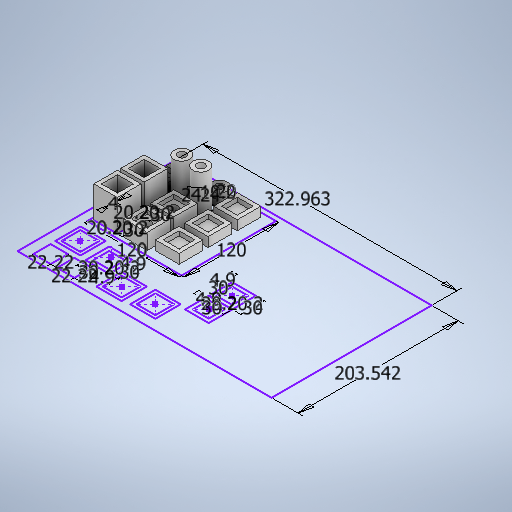
# Autodesk Inventor part: zxie2
Saved by Autodesk Inventor 2025.1 (Build 291241000, 241)
## iProperties
Created: 2024-10-25
Part Number: zxie2
Material: 一般
Document SubType Name: Modeling
Designer: youtian
Density: 1 g/cm^3
Appearance: 預設
Author: youtian
Autodesk Inventor part; units mm, degrees
ref_plane "YZ Plane" through (0, 0, 0) normal (1, 0, 0) x (0, 1, 0)
ref_plane "XZ Plane" through (0, 0, 0) normal (0, 1, 0) x (-1, 0, 0)
ref_plane "XY Plane" through (0, 0, 0) normal (0, 0, 1) x (1, 0, 0)
sketch "草圖1" plane through (0, 0, 0) normal (0, 1, 0) x (-1, 0, 0)
  circle A0 centre (0, 0) radius 5.1
  circle A1 centre (0, 0) radius 10
  line L0 (0, 0) -> (-26.517, 0)
  line L1 (0, 0) -> (0, 28.4195)
  circle A2 centre (-24, 0) radius 5.1
  circle A3 centre (-24, 0) radius 10
  circle A4 centre (0, 24) radius 5.1
  circle A5 centre (0, 24) radius 10
  circle A6 centre (-24, 24) radius 5.1
  circle A7 centre (-24, 24) radius 10
  dimension "d6" = 24
  dimension "d9" = 24
  dimension "d137" = 10.2
  dimension "d138" = 20
  constraints: 8 centre point, 5 coincident, 4 end point, 2 horizontal, 2 vertical, 12 other
  measures "d6" distance of A0.centre A2.centre
  measures "d9" distance of A0.centre A4.centre
  measures "d137" diameter of A0
  measures "d138" diameter of A1
extrude "擠出1" add sketch "草圖1" along normal blind 15 contours A0 L1 A1 L0 | A0 L0 A1 L1 | A3
extrude "擠出2" add sketch "草圖1" along normal blind 50 contours A5 | A7
sketch "草圖2" plane through (0, 0, 0) normal (0, 1, 0) x (-1, 0, 0)
  line L0 (-38.8717, -7.5692) -> (-68.8717, -7.5692)
  line L1 (-68.8717, -7.5692) -> (-68.8717, 22.4308)
  line L2 (-68.8717, 22.4308) -> (-38.8717, 22.4308)
  line L3 (-38.8717, 22.4308) -> (-38.8717, -7.5692)
  point P0 (0, 0)
  dimension "d14" = 30
  dimension "d15" = 30
  constraints: 8 end point, 2 parallel, 1 horizontal, 1 perpendicular
  measures "d14" distance of L1.end L2.end
  measures "d15" distance of L0.end L1.end
extrude "擠出3" add sketch "草圖2" along normal blind 12
sketch "草圖3" plane through (0, 12, 0) normal (0, 1, 0) x (1, 0, 0)
  line L0 (68.8717, -22.4308) -> (68.8717, 7.5692) projected
  line L1 (68.8717, 7.5692) -> (36.4675, -24.4308)
  line L2 (68.8717, 7.5692) -> (38.8717, 7.5692) projected
  line L3 (38.8717, 7.5692) -> (68.8717, -22.4308)
  line L4 (43.8717, 2.5692) -> (63.8717, 2.5692)
  line L5 (63.8717, 2.5692) -> (63.8717, -17.4308)
  line L6 (63.8717, -17.4308) -> (43.8717, -17.4308)
  line L7 (43.8717, -17.4308) -> (43.8717, 2.5692)
  line L8 (43.8717, 2.5692) -> (63.8717, -17.4308) construction
  line L9 (63.8717, 2.5692) -> (43.8717, -17.4308) construction
  point P0 (0, 0)
  point P1 (53.8717, -7.4308)
  dimension "d18" = 20
  dimension "d19" = 20
  constraints: 16 end point, 3 midpoint, 2 parallel, 1 horizontal, 1 perpendicular
  measures "d18" distance of L5.end L6.end
  measures "d19" distance of L4.end L5.end
extrude "擠出4" cut sketch "草圖3" against normal blind 5.6 contours L6 L7 L1 L3 | L3 L1 L4 L5 | L1 L3 L4 | L1 L7 L3
pattern_linear "矩形陣列1" count 3 spacing 37 along (0, 0, 1) of "擠出3", "擠出4"
sketch "草圖4" plane through (0, 0, 0) normal (0, 1, 0) x (-1, 0, 0)
  line L0 (-33.3892, 37.5706) -> (-3.3892, 37.5706)
  line L1 (-3.3892, 37.5706) -> (-3.3892, 67.5706)
  line L2 (-3.3892, 67.5706) -> (-33.3892, 67.5706)
  line L3 (-33.3892, 67.5706) -> (-33.3892, 37.5706)
  circle A0 centre (-18.3892, 52.5706) radius 5.1
  point P0 (0, 0)
  point P1 (-18.3892, 67.5706)
  point P2 (-3.3892, 52.5706)
  dimension "d28" = 30
  dimension "d29" = 30
  dimension "d30" = 10.2
  dimension "d141" = 15
  dimension "d142" = 15
  constraints: 8 end point, 2 midpoint, 2 parallel, 1 centre point, 1 horizontal, 1 perpendicular
  measures "d28" distance of L2.end L1.end
  measures "d29" distance of L1.end L0.end
  measures "d30" diameter of A0
  measures "d141" distance of point (-18.389, 67.571) A0.centre
  measures "d142" distance of A0.centre point (-3.389, 52.571)
extrude "擠出5" add sketch "草圖4" along normal blind 15
sketch "草圖5" plane through (0, 15, 0) normal (0, 1, 0) x (1, 0, 0)
  line L0 (3.3892, -37.5706) -> (3.3892, -67.5706) projected
  line L1 (3.3892, -67.5706) -> (33.3892, -67.5706) projected
  line L2 (3.3892, -37.5706) -> (33.3892, -37.5706)
  line L3 (33.3892, -37.5706) -> (33.3892, -67.5706)
  line L4 (33.3892, -67.5706) -> (3.3892, -67.5706)
  line L5 (3.3892, -67.5706) -> (3.3892, -37.5706)
  line L6 (8.2892, -42.4706) -> (28.4892, -42.4706)
  line L7 (28.4892, -42.4706) -> (28.4892, -62.6706)
  line L8 (28.4892, -62.6706) -> (8.2892, -62.6706)
  line L9 (8.2892, -62.6706) -> (8.2892, -42.4706)
  circle A0 centre (18.3892, -52.5706) radius 5.1 projected
  line L10 (8.2892, -42.4706) -> (28.4892, -62.6706) construction
  line L11 (28.4892, -42.4706) -> (8.2892, -62.6706) construction
  point P0 (0, 0)
  dimension "d33" = 20.2
  dimension "d34" = 20.2
  constraints: 20 end point, 4 parallel, 2 horizontal, 2 midpoint, 2 perpendicular
  measures "d33" distance of L7.end L8.end
  measures "d34" distance of L6.end L7.end
extrude "擠出6" add sketch "草圖5" along normal blind 5 contours L2 L3 L1 L0
pattern_linear "矩形陣列2" count 2 spacing 34 along (0, 0, 1) of "擠出5", "擠出6"
sketch "草圖6" plane through (0, 0, 0) normal (0, 1, 0) x (-1, 0, 0)
  point P0 (0, 0)
sketch "草圖9" plane through (0, 0, 0) normal (0, 1, 0) x (-1, 0, 0)
  line L0 (-122.3877, 82.2379) -> (-152.3877, 82.2379)
  line L1 (-152.3877, 82.2379) -> (-152.3877, 112.2379)
  line L2 (-152.3877, 112.2379) -> (-122.3877, 112.2379)
  line L3 (-122.3877, 112.2379) -> (-122.3877, 82.2379)
  line L4 (-127.2877, 87.1379) -> (-147.4877, 87.1379)
  line L5 (-147.4877, 87.1379) -> (-147.4877, 107.3379)
  line L6 (-147.4877, 107.3379) -> (-127.2877, 107.3379)
  line L7 (-127.2877, 107.3379) -> (-127.2877, 87.1379)
  line L8 (-127.2877, 87.1379) -> (-147.4877, 107.3379) construction
  line L9 (-147.4877, 87.1379) -> (-127.2877, 107.3379) construction
  line L10 (-122.3877, 112.2379) -> (-152.3877, 112.2379)
  line L11 (-152.3877, 112.2379) -> (-152.3877, 142.2379)
  line L12 (-152.3877, 142.2379) -> (-122.3877, 142.2379)
  line L13 (-122.3877, 142.2379) -> (-122.3877, 112.2379)
  line L14 (-127.2877, 117.1379) -> (-147.4877, 117.1379)
  line L15 (-147.4877, 117.1379) -> (-147.4877, 137.3379)
  line L16 (-147.4877, 137.3379) -> (-127.2877, 137.3379)
  line L17 (-127.2877, 137.3379) -> (-127.2877, 117.1379)
  line L18 (-127.2877, 117.1379) -> (-147.4877, 137.3379) construction
  line L19 (-147.4877, 117.1379) -> (-127.2877, 137.3379) construction
  line L20 (-4.8445, 121.2719) -> (-34.8445, 121.2719)
  line L21 (-34.8445, 121.2719) -> (-34.8445, 151.2719)
  line L22 (-34.8445, 151.2719) -> (-4.8445, 151.2719)
  line L23 (-4.8445, 151.2719) -> (-4.8445, 121.2719)
  line L24 (-9.7445, 126.1719) -> (-29.9445, 126.1719)
  line L25 (-29.9445, 126.1719) -> (-29.9445, 146.3719)
  line L26 (-29.9445, 146.3719) -> (-9.7445, 146.3719)
  line L27 (-9.7445, 146.3719) -> (-9.7445, 126.1719)
  line L28 (-5.9445, 119.5982) -> (-29.9445, 143.5982) construction
  line L29 (-29.9445, 119.5982) -> (-5.9445, 143.5982) construction
  line L30 (30.8593, 41.0028) -> (6.8593, 65.0028) construction
  line L31 (6.8593, 41.0028) -> (30.8593, 65.0028) construction
  line L32 (35.5473, 117.4293) -> (3.5473, 117.4293)
  line L33 (31.5472, 121.4294) -> (7.5472, 121.4294)
  line L34 (7.5472, 121.4294) -> (7.5472, 145.4294)
  line L35 (3.5473, 117.4293) -> (3.5473, 149.4293)
  line L36 (7.5472, 145.4294) -> (31.5472, 145.4294)
  line L37 (31.5472, 121.4294) -> (7.5472, 145.4294) construction
  line L38 (7.5472, 121.4294) -> (31.5472, 145.4294) construction
  line L39 (3.5473, 149.4293) -> (35.5473, 149.4293)
  line L40 (31.5472, 145.4294) -> (31.5472, 121.4294)
  line L41 (35.5473, 149.4293) -> (35.5473, 117.4293)
  line L42 (-40.805, 141.4327) -> (-72.805, 141.4327)
  line L43 (-44.805, 145.4328) -> (-68.805, 145.4328)
  line L44 (-68.805, 145.4328) -> (-68.805, 169.4328)
  line L45 (-72.805, 141.4327) -> (-72.805, 173.4327)
  line L46 (-68.805, 169.4328) -> (-44.805, 169.4328)
  line L47 (-44.805, 145.4328) -> (-68.805, 169.4328) construction
  line L48 (-68.805, 145.4328) -> (-44.805, 169.4328) construction
  line L49 (-72.805, 173.4327) -> (-40.805, 173.4327)
  line L50 (-44.805, 169.4328) -> (-44.805, 145.4328)
  line L51 (-40.805, 173.4327) -> (-40.805, 141.4327)
  line L52 (-81.8163, 139.4435) -> (-113.8163, 139.4435)
  line L53 (-85.8164, 143.4436) -> (-109.8164, 143.4436)
  line L54 (-109.8164, 143.4436) -> (-109.8164, 167.4436)
  line L55 (-113.8163, 139.4435) -> (-113.8163, 171.4435)
  line L56 (-109.8164, 167.4436) -> (-85.8164, 167.4436)
  line L57 (-85.8164, 143.4436) -> (-109.8164, 167.4436) construction
  line L58 (-109.8164, 143.4436) -> (-85.8164, 167.4436) construction
  line L59 (-113.8163, 171.4435) -> (-81.8163, 171.4435)
  line L60 (-85.8164, 167.4436) -> (-85.8164, 143.4436)
  line L61 (-81.8163, 171.4435) -> (-81.8163, 139.4435)
  line L62 (28.9593, 42.9028) -> (8.7593, 42.9028)
  line L63 (8.7593, 42.9028) -> (8.7593, 63.1028)
  line L64 (8.7593, 63.1028) -> (28.9593, 63.1028)
  line L65 (28.9593, 63.1028) -> (28.9593, 42.9028)
  line L66 (28.9593, 42.9028) -> (8.7593, 63.1028) construction
  line L67 (8.7593, 42.9028) -> (28.9593, 63.1028) construction
  line L68 (33.8593, 38.0028) -> (3.8593, 38.0028)
  line L69 (3.8593, 38.0028) -> (3.8593, 68.0028)
  line L70 (3.8593, 68.0028) -> (33.8593, 68.0028)
  line L71 (33.8593, 68.0028) -> (33.8593, 38.0028)
  line L72 (33.8593, 38.0028) -> (3.8593, 68.0028) construction
  line L73 (3.8593, 38.0028) -> (33.8593, 68.0028) construction
  line L74 (6.8593, 78.0206) -> (30.8593, 102.0206) construction
  line L75 (30.8593, 78.0206) -> (6.8593, 102.0206) construction
  line L76 (28.9593, 76.9028) -> (8.7593, 76.9028)
  line L77 (8.7593, 76.9028) -> (8.7593, 97.1028)
  line L78 (8.7593, 97.1028) -> (28.9593, 97.1028)
  line L79 (28.9593, 97.1028) -> (28.9593, 76.9028)
  line L80 (28.9593, 76.9028) -> (8.7593, 97.1028) construction
  line L81 (8.7593, 76.9028) -> (28.9593, 97.1028) construction
  line L82 (33.8593, 72.0028) -> (3.8593, 72.0028)
  line L83 (3.8593, 72.0028) -> (3.8593, 102.0028)
  line L84 (3.8593, 102.0028) -> (33.8593, 102.0028)
  line L85 (33.8593, 102.0028) -> (33.8593, 72.0028)
  line L86 (33.8593, 72.0028) -> (3.8593, 102.0028) construction
  line L87 (3.8593, 72.0028) -> (33.8593, 102.0028) construction
  point P0 (0, 0)
  point P1 (-137.3877, 97.2379)
  point P2 (-137.3877, 127.2379)
  point P3 (-17.9445, 131.5982)
  point P4 (18.8593, 53.0028)
  point P5 (19.5472, 133.4294)
  point P6 (-56.805, 157.4328)
  point P7 (-97.8164, 155.4436)
  point P8 (30.8593, 102.0206)
  point P9 (30.8593, 78.0206)
  point P10 (6.8593, 78.0206)
  point P11 (6.8593, 102.0206)
  point P12 (18.8593, 87.0028)
  dimension "d73" = 50.747
  dimension "d54" = 30
  dimension "d55" = 30
  dimension "d56" = 20.2
  dimension "d57" = 20.2
  dimension "d60" = 30
  dimension "d69" = 30
  dimension "d70" = 30
  dimension "d71" = 20.2
  dimension "d72" = 20.2
  dimension "d139" = 4.9
  dimension "d140" = 4.9
  dimension "d143" = 4.9
  dimension "d144" = 4.9
  dimension "d145" = 20.2
  dimension "d146" = 20.2
  dimension "d148" = 30
  dimension "d153" = 20.2
  dimension "d154" = 20.2
  dimension "d155" = 30
  dimension "d158" = 4
  constraints: 172 end point, 16 parallel, 12 midpoint, 8 horizontal, 8 perpendicular, 2 vertical, 1 collinear, 24 other
  measures "d54" distance of L1.end L2.end
  measures "d55" distance of L0.end L1.end
  measures "d56" distance of L5.end L6.end
  measures "d57" distance of L4.end L5.end
  measures "d60" distance of L0.start L10.start
  measures "d69" distance of L22.start L22.end
  measures "d70" distance of L20.end L22.start
  measures "d71" distance of L26.start L26.end
  measures "d72" distance of L24.end L26.start
  measures "d139" horizontal distance of L24.end L20.end
  measures "d140" horizontal distance of L26.start L22.start
  measures "d143" horizontal distance of L4.start L0.start
  measures "d144" horizontal distance of L6.end L2.end
  measures "d145" distance of L63.end L64.end
  measures "d146" distance of L62.end L63.end
  measures "d148" distance of L68.end L69.end
  measures "d153" distance of L77.end L78.end
  measures "d154" distance of L77.start L77.end
  measures "d155" distance of L82.end L84.start
  measures "d158" distance of L82.start L70.end
extrude "擠出10" [suppressed]
sketch "草圖10" plane through (0, 0, 0) normal (0, 1, 0) x (-1, 0, 0)
  line L0 (48.2716, 184.5725) -> (-274.6912, 184.5725)
  line L1 (-274.6912, 184.5725) -> (-274.6912, -18.9692)
  line L2 (-274.6912, -18.9692) -> (48.2716, -18.9692)
  line L3 (48.2716, -18.9692) -> (48.2716, 184.5725)
  point P0 (0, 0)
  dimension "d99" = 322.9628
  dimension "d100" = 203.5417
  constraints: 8 end point, 2 parallel, 1 horizontal, 1 perpendicular
  measures "d99" distance of L1.end L2.end
  measures "d100" distance of L0.end L1.end
sketch "草圖11" plane through (0, 0, 0) normal (0, 1, 0) x (-1, 0, 0)
  line L0 (35.0654, 155.7952) -> (13.0654, 155.7952)
  line L1 (13.0654, 155.7952) -> (13.0654, 177.7952)
  line L2 (13.0654, 177.7952) -> (35.0654, 177.7952)
  line L3 (35.0654, 177.7952) -> (35.0654, 155.7952)
  line L4 (4.7905, 155.7952) -> (-17.2095, 155.7952)
  line L5 (-17.2095, 155.7952) -> (-17.2095, 177.7952)
  line L6 (-17.2095, 177.7952) -> (4.7905, 177.7952)
  line L7 (4.7905, 177.7952) -> (4.7905, 155.7952)
  point P0 (0, 0)
  dimension "d101" = 22
  dimension "d102" = 22
  dimension "d103" = 22
  dimension "d104" = 22
  constraints: 16 end point, 4 parallel, 2 horizontal, 2 perpendicular
  measures "d101" distance of L1.end L2.end
  measures "d102" distance of L0.end L1.end
  measures "d103" distance of L5.end L6.end
  measures "d104" distance of L4.end L5.end
sketch "草圖12" plane through (0, 0, 0) normal (0, 1, 0) x (-1, 0, 0)
  line L0 (16.0858, 34.2244) -> (36.0858, 34.2244)
  line L1 (36.0858, 34.2244) -> (36.0858, 14.2244)
  line L2 (36.0858, 14.2244) -> (16.0858, 14.2244)
  line L3 (16.0858, 14.2244) -> (16.0858, 34.2244)
  line L4 (16.0552, 8.0877) -> (36.0552, 8.0877)
  line L5 (36.0552, 8.0877) -> (36.0552, -11.9123)
  line L6 (36.0552, -11.9123) -> (16.0552, -11.9123)
  line L7 (16.0552, -11.9123) -> (16.0552, 8.0877)
  point P0 (0, 0)
  dimension "d105" = 20
  dimension "d106" = 20
  dimension "d107" = 20
  dimension "d108" = 20
  constraints: 16 end point, 4 parallel, 2 horizontal, 2 perpendicular
  measures "d105" distance of L1.end L2.end
  measures "d106" distance of L0.end L1.end
  measures "d107" distance of L5.end L6.end
  measures "d108" distance of L4.end L5.end
extrude "擠出12" add sketch "草圖12" along normal blind 12
sketch "草圖13" plane through (0, 12, 0) normal (0, 1, 0) x (1, 0, 0)
  line L0 (-16.0552, 11.9123) -> (-36.0552, 11.9123) projected
  line L1 (-36.0552, -8.0877) -> (-16.0552, -8.0877) projected
  line L2 (-36.0552, 11.9123) -> (-16.0552, -8.0877)
  line L3 (-36.0858, -14.2244) -> (-36.0858, -34.2244) projected
  line L4 (-36.0858, -34.2244) -> (-16.0858, -34.2244) projected
  line L5 (-36.0858, -14.2244) -> (-16.0858, -34.2244)
  line L6 (-13.0654, -155.7952) -> (-35.0654, -155.7952) projected
  line L7 (-35.0654, -177.7952) -> (-13.0654, -177.7952) projected
  line L8 (-35.0654, -155.7952) -> (-13.0654, -177.7952)
  line L9 (-4.7905, -177.7952) -> (17.2095, -177.7952) projected
  line L10 (-4.7905, -155.7952) -> (17.2095, -177.7952)
  line L11 (-31.0654, -159.7952) -> (-17.0654, -159.7952)
  line L12 (-17.0654, -159.7952) -> (-17.0654, -173.7952)
  line L13 (-17.0654, -173.7952) -> (-31.0654, -173.7952)
  line L14 (-31.0654, -173.7952) -> (-31.0654, -159.7952)
  line L15 (-31.0654, -159.7952) -> (-17.0654, -173.7952) construction
  line L16 (-17.0654, -159.7952) -> (-31.0654, -173.7952) construction
  line L17 (-0.7905, -173.7952) -> (13.2095, -173.7952)
  line L18 (13.2095, -173.7952) -> (13.2095, -159.7952)
  line L19 (13.2095, -159.7952) -> (-0.7905, -159.7952)
  line L20 (-0.7905, -159.7952) -> (-0.7905, -173.7952)
  line L21 (-0.7905, -173.7952) -> (13.2095, -159.7952) construction
  line L22 (13.2095, -173.7952) -> (-0.7905, -159.7952) construction
  line L23 (-31.1552, 7.0123) -> (-20.9552, 7.0123)
  line L24 (-20.9552, 7.0123) -> (-20.9552, -3.1877)
  line L25 (-20.9552, -3.1877) -> (-31.1552, -3.1877)
  line L26 (-31.1552, -3.1877) -> (-31.1552, 7.0123)
  line L27 (-31.1552, 7.0123) -> (-20.9552, -3.1877) construction
  line L28 (-20.9552, 7.0123) -> (-31.1552, -3.1877) construction
  line L29 (-31.1858, -29.3244) -> (-20.9858, -29.3244)
  line L30 (-20.9858, -29.3244) -> (-20.9858, -19.1244)
  line L31 (-20.9858, -19.1244) -> (-31.1858, -19.1244)
  line L32 (-31.1858, -19.1244) -> (-31.1858, -29.3244)
  line L33 (-31.1858, -29.3244) -> (-20.9858, -19.1244) construction
  line L34 (-20.9858, -29.3244) -> (-31.1858, -19.1244) construction
  point P0 (0, 0)
  point P1 (-24.0654, -166.7952)
  point P2 (6.2095, -166.7952)
  point P3 (-26.0552, 1.9123)
  point P4 (-26.0858, -24.2244)
  dimension "d113" = 14
  dimension "d114" = 14
  dimension "d115" = 14
  dimension "d116" = 14
  dimension "d117" = 10.2
  dimension "d118" = 10.2
  dimension "d119" = 10.2
  dimension "d120" = 10.2
  constraints: 56 end point, 12 midpoint, 8 parallel, 4 horizontal, 4 perpendicular
  measures "d113" distance of L12.end L13.end
  measures "d114" distance of L11.end L12.end
  measures "d115" distance of L19.end L18.end
  measures "d116" distance of L18.end L17.end
  measures "d117" distance of L24.end L25.end
  measures "d118" distance of L23.end L24.end
  measures "d119" distance of L31.end L30.end
  measures "d120" distance of L30.end L29.end
extrude "擠出13" cut sketch "草圖13" against normal blind 5.6 contours L23 L24 L2 | L2 L25 L26 | L31 L30 L5 | L5 L29 L32 | L11 L12 L8 | L8 L13 L14 | L19 L18 L10 | L10 L17 L20
sketch "草圖15" plane through (0, 0, 0) normal (0, 1, 0) x (-1, 0, 0)
  line L0 (37.1328, -12.8546) -> (-82.8672, -12.8546)
  line L1 (-82.8672, -12.8546) -> (-82.8672, 107.1454)
  line L2 (-82.8672, 107.1454) -> (37.1328, 107.1454)
  line L3 (37.1328, 107.1454) -> (37.1328, -12.8546)
  point P0 (0, 0)
  dimension "d135" = 120
  dimension "d136" = 120
  constraints: 8 end point, 2 parallel, 1 horizontal, 1 perpendicular
  measures "d135" distance of L1.end L2.end
  measures "d136" distance of L0.end L1.end
extrude "擠出15" add sketch "草圖9" along normal blind 40 contours L68 L69 L70 L71 | L82 L83 L84 L85
